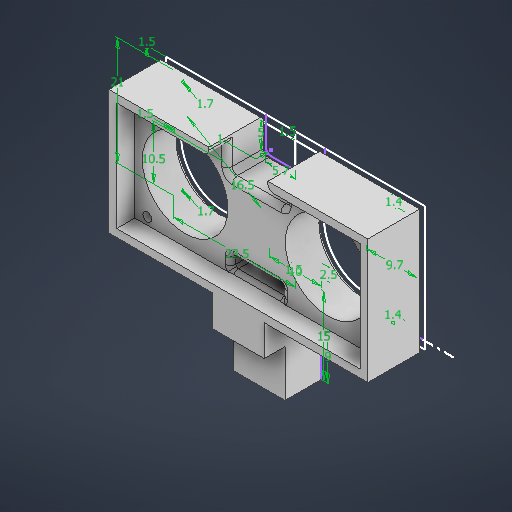
# Autodesk Inventor part: us-sensor-mount_backup
Saved by Autodesk Inventor 2026.2 (Build 302298010, 298A)
## iProperties
Created: 2026-03-09
Part Number: us-sensor-mount_backup
Material: Generic
Document SubType Name: Modeling
Designer: david
Density: 1 g/cm^3
Appearance: Default
Author: david
Autodesk Inventor part; units mm, degrees
ref_plane "YZ Plane" through (0, 0, 0) normal (1, 0, 0) x (0, 1, 0)
ref_plane "XZ Plane" through (0, 0, 0) normal (0, 1, 0) x (-1, 0, 0)
ref_plane "XY Plane" through (0, 0, 0) normal (0, 0, 1) x (1, 0, 0)
sketch "Block1" plane through (0, 0, 0) normal (0, 0, 1) x (1, 0, 0)
  line L0 (-4.7991, 20.985) -> (-24.4491, 20.985)
  line L1 (-24.4491, 20.985) -> (-24.4491, 0.985)
  line L2 (-4.6891, 3.825) -> (-6.8291, 3.825)
  line L3 (-4.6891, 1.685) -> (-4.6891, 3.825)
  line L4 (-6.8291, 1.685) -> (-4.6891, 1.685)
  line L5 (-6.8291, 3.825) -> (-6.8291, 1.685)
  line L6 (-2.1491, 3.825) -> (-4.2891, 3.825)
  line L7 (-2.1491, 1.685) -> (-2.1491, 3.825)
  line L8 (-1.9491, 16.485) -> (-6.9491, 16.485)
  line L9 (-1.9491, 0.985) -> (-1.9491, 20.985)
  line L10 (-7.9491, 17.485) -> (-7.9491, 20.985)
  circle A0 centre (-23.0491, 2.385) radius 0.85
  line L11 (-24.4491, 0.985) -> (-1.9491, 0.985)
  circle A1 centre (-14.7491, 10.985) radius 8.25
  line L12 (-24.4491, 20.985) -> (-24.4491, 0.985)
  circle A2 centre (-23.0491, 19.585) radius 0.85
  line L13 (-1.9491, 20.985) -> (-24.4491, 20.985)
  line L14 (-4.2891, 3.825) -> (-4.2891, 1.685)
  line L15 (-4.2891, 1.685) -> (-2.1491, 1.685)
  line L16 (-1.9491, 3.825) -> (-1.9491, 1.685)
  line L17 (-6.8291, 1.685) -> (-6.8291, 3.825)
  line L18 (-1.9491, 1.685) -> (-6.8291, 1.685)
  line L19 (-6.8291, 3.825) -> (-1.9491, 3.825)
  arc A3 (-7.9491, 17.485) -> (-6.9491, 16.485) centre (-6.9491, 17.485) ccw
  point P0 (-8.1512, 8.999)
  point P1 (-1.9491, 10.985)
  point P2 (-7.9491, 16.485)
  dimension "d1" = 16.5
  dimension "d2" = 1.7
  dimension "d3" = 1.7
  dimension "d4" = 6
  dimension "d5" = 4.5
  dimension "d6" = 1
  measures "d1" diameter of A1
  measures "d2" diameter of A2
  measures "d3" diameter of A0
  measures "d4" distance of L8.start point (-7.949, 16.485)
  measures "d5" distance of point (-7.949, 16.485) L10.end
  measures "d6" radius of A3
sketch "Sketch1" plane through (0, 0, 0) normal (0, 0, 1) x (1, 0, 0)
  line L0 (0, 14.2564) -> (0, -13.7436)
  line L1 (-32.4077, 0) -> (30.5923, 0)
  line L2 (2.55, 21) -> (23.5, 21)
  line L3 (23.5, 21) -> (23.5, 0)
  line L4 (0, 16) -> (4.7, 16)
  line L5 (0, 0) -> (0, 21)
  line L6 (5.7, 17) -> (5.7, 21)
  circle A0 centre (21.1, 1.4) radius 0.85
  line L7 (23.5, 0) -> (0, 0)
  circle A1 centre (13.8, 10.5) radius 8.25
  line L8 (23.5, 21) -> (23.5, 0)
  circle A2 centre (21.1, 19.6) radius 0.85
  line L9 (0, 21) -> (23.5, 21)
  arc A3 (4.7, 16) -> (5.7, 17) centre (4.7, 17) ccw
  arc A4 (-5.7, 17) -> (-4.7, 16) centre (-4.7, 17) ccw
  line L10 (-2.55, 21) -> (-23.5, 21)
  line L11 (-23.5, 21) -> (-23.5, 0)
  circle A5 centre (-13.8, 10.5) radius 8.25
  circle A6 centre (-21.1, 19.6) radius 0.85
  circle A7 centre (-21.1, 1.4) radius 0.85
  line L12 (0, 21) -> (-23.5, 21)
  line L13 (-23.5, 21) -> (-23.5, 0)
  line L14 (-23.5, 0) -> (0, 0)
  line L15 (0, 0) -> (0, 21)
  line L16 (0, 16) -> (-4.7, 16)
  line L17 (-5.7, 17) -> (-5.7, 21)
  line L18 (0, 2.84) -> (0, 0.7)
  line L19 (-5, 3.02) -> (5, 3.02)
  line L20 (5, 3.02) -> (5, 0.52)
  line L21 (5, 0.52) -> (-5, 0.52)
  line L22 (-5, 0.52) -> (-5, 3.02)
  line L23 (-5, 3.02) -> (5, 0.52) construction
  line L24 (5, 3.02) -> (-5, 0.52) construction
  line L25 (0, 21) -> (0, 22.5)
  line L26 (0, 0) -> (0, -1.5)
  line L27 (0, -1.5) -> (-25, -1.5)
  line L28 (-25, -1.5) -> (-25, 22.5)
  line L29 (-25, 22.5) -> (0, 22.5)
  line L30 (0, 22.5) -> (0, -1.5)
  arc A8 (4.7, 16) -> (5.7, 17) centre (4.7, 17) ccw
  line L31 (2.55, 21) -> (23.5, 21)
  line L32 (23.5, 21) -> (23.5, 0)
  circle A9 centre (13.8, 10.5) radius 8.25
  circle A10 centre (21.1, 19.6) radius 0.85
  circle A11 centre (21.1, 1.4) radius 0.85
  line L33 (0, 21) -> (23.5, 21)
  line L34 (23.5, 21) -> (23.5, 0)
  line L35 (23.5, 0) -> (0, 0)
  line L36 (0, 16) -> (4.7, 16)
  line L37 (5.7, 17) -> (5.7, 21)
  line L38 (5, 0.52) -> (5, 3.02)
  line L39 (23.5, 0) -> (24.5, 0)
  line L40 (0, -1.5) -> (25, -1.5)
  line L41 (25, -1.5) -> (25, 22.5)
  line L42 (25, 22.5) -> (0, 22.5)
  line L43 (-5, -1.5) -> (5, -1.5)
  line L44 (5, -1.5) -> (5, -16.5)
  line L45 (5, -16.5) -> (-5, -16.5)
  line L46 (-5, -16.5) -> (-5, -1.5)
  line L47 (-5, -16.5) -> (5, -16.5)
  line L48 (5, -16.5) -> (5, -7.5)
  line L49 (5, -7.5) -> (-5, -7.5)
  line L50 (-5, -7.5) -> (-5, -16.5)
  line L51 (-5.7, 21) -> (-5.7, 22.5)
  line L52 (5.7, 21) -> (5.7, 22.5)
  point P0 (0, 10)
  point P1 (5.7, 16)
  point P2 (0, 10)
  point P3 (-5.7, 16)
  point P4 (0, 1.77)
  point P5 (-5.7, 21)
  point P6 (23.5, 0)
  point P7 (5.7, 21)
  dimension "d7" = 16.5
  dimension "d8" = 1.7
  dimension "d9" = 1.7
  dimension "d10" = 5.7
  dimension "d11" = 5
  dimension "d12" = 1
  dimension "d13" = 10
  dimension "d14" = 2.5
  dimension "d15" = 1.5
  dimension "d16" = 1.5
  dimension "d18" = 15
  dimension "d19" = 9
  dimension "d20" = 23.5
  dimension "d21" = 1.5
  dimension "d22" = 1.5
  dimension "d23" = 21
  dimension "d43" = 1.4
  dimension "d44" = 1.4
  dimension "d45" = 9.7
  dimension "d49" = 10.5
  constraints: 106 end point, 21 symmetric about line, 20 point on line, 12 centre point, 8 parallel, 7 perpendicular, 6 point on circle, 5 horizontal, 4 collinear, 3 midpoint, 2 tangent, 2 vertical, 8 other
  measures "d7" diameter of A5
  measures "d8" diameter of A6
  measures "d9" diameter of A7
  measures "d10" distance of L16.start point (-5.7, 16)
  measures "d11" distance of point (-5.7, 16) L17.end
  measures "d12" radius of A4
  measures "d13" distance of L20.end L21.end
  measures "d14" distance of L19.end L20.end
  measures "d15" distance of L12.start L25.end
  measures "d16" distance of L14.end L26.end
  measures "d18" distance of L43.end L44.end
  measures "d19" distance of L48.end L47.end
  measures "d20" distance of L11.end L14.end
  measures "d21" distance between parallel lines of L11 L28
  measures "d22" distance between parallel lines of L29 L10
  measures "d23" distance of L10.end L11.end
  measures "d43" distance from line of L2 A2.centre
  measures "d44" distance from line of A0.centre L7
  measures "d45" distance from line of L3 A9.centre
  measures "d49" distance from line of L14 A5.centre
extrude "Extrusion1" add sketch "Sketch1" along normal blind 7.5 contours L19 L22 L21 L0 L1 L11 L10 L17 A4 L16 L5 | L0 L5 L4 A3 L6 L2 L3 L1 L21 L20 L19
extrude "Extrusion2" add sketch "Sketch1" along normal blind 11 contours L1 L41 L40 L0 | L0 L27 L28 L1 | L1 L28 L29 L51 L10 L11 | L3 L2 L52 L42 L41 L1 | L25 L42 L52 L2 L9 | L12 L10 L51 L29 L25
extrude "Extrusion3" add sketch "Sketch1" along normal blind 11 contours L40 L44 L49 L0 | L0 L49 L46 L27
extrude "Extrusion4" add sketch "Sketch1" along normal blind 7 contours L49 L44 L45 L46
chamfer "Chamfer1" distance 1 angle 45 7 edges at (5.55, 10.5, 0) (-22.05, 10.5, 0) (-15, -1.5, 0) (15, -1.5, 0) (25, 10.5, 0) (-25, 10.5, 0) (0, 22.5, 0)
chamfer "Chamfer2" distance 0.4 angle 45 4 edges at (-21.95, 19.6, 0) (20.25, 19.6, 0) (20.25, 1.4, 0) (-21.95, 1.4, 0)
fillet "Fillet1" radius 0.5 1 edges at (-5, 3.02, 3.75)
fillet "Fillet2" radius 0.5 1 edges at (5, 3.02, 3.75)
fillet "Fillet3" radius 0.5 2 edges at (5, 0.52, 3.75) (-5, 0.52, 3.75)
extrude "Extrusion5" cut sketch "Sketch1" along normal blind 15 contours L25 L42 L52 L2 L9 | L12 L10 L51 L29 L25
chamfer "Chamfer3" distance 0.5 angle 45 5 edges at (0, 16, 0) (-5.4071, 16.2929, 0) (-5.7, 19.25, 0) (5.4071, 16.2929, 0) (5.7, 19.25, 0)
fillet "Fillet4" radius 1 15 edges at (-5.4071, 16.2929, 7.5) (-5.7, 19, 7.5) (5.4071, 16.2929, 7.5) (5.7, 19, 7.5) (0, 16, 7.5) (-5.7, 21, 9.25) (5.7, 21, 9.25) (4.8536, 2.8736, 7.5) (5, 1.77, 7.5) (4.8536, 0.6664, 7.5) (0, 0.52, 7.5) (-4.8536, 0.6664, 7.5) (-5, 1.77, 7.5) (-4.8536, 2.8736, 7.5) (0, 3.02, 7.5)
body "Solid1"
